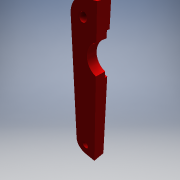
# Autodesk Inventor part: Carro XY_trava_A
Saved by Autodesk Inventor 2016 (Build 200138000, 138)
## iProperties
Created: 2016-08-11
Part Number: Carro XY_trava_A
Material: ABS Plastic
Document SubType Name: Modeling
Designer: Waldo
Density: 1.06 g/cm^3
Appearance: Smooth - White
Author: Waldo
Autodesk Inventor part; units mm, degrees
ref_plane "YZ Plane" through (0, 0, 0) normal (1, 0, 0) x (0, 1, 0)
ref_plane "XZ Plane" through (0, 0, 0) normal (0, 1, 0) x (-1, 0, 0)
ref_plane "XY Plane" through (0, 0, 0) normal (0, 0, 1) x (1, 0, 0)
sketch "Sketch1" plane through (0, 0, 0) normal (0, 1, 0) x (-1, 0, 0)
  line L0 (14.0376, 28.5915) -> (4.0376, 28.5915)
  line L1 (4.0376, 28.5915) -> (4.0376, -31.4085)
  line L2 (4.0376, -31.4085) -> (14.0376, -31.4085)
  line L3 (14.0376, -31.4085) -> (14.0376, 28.5915)
  point P0 (0, 0)
  dimension "d0" = 60
  dimension "d1" = 10
  constraints: 8 end point, 2 parallel, 1 horizontal, 1 perpendicular
  measures "d0" distance of L2.end L0.start
  measures "d1" distance of L0.start L0.end
extrude "Extrusion1" add sketch "Sketch1" along normal blind 5.2
sketch "Sketch2" plane through (0, 0, 0) normal (0, -1, 0) x (1, 0, 0)
  arc A0 (-14.0376, -26.4085) -> (-9.0376, -31.4085) centre (-9.0376, -26.4085) ccw projected
  arc A1 (-9.0376, 28.5915) -> (-14.0376, 23.5915) centre (-9.0376, 23.5915) ccw projected
  circle A2 centre (-9.0376, -26.4085) radius 1.5 projected
  circle A3 centre (-9.0376, 23.5915) radius 1.5 projected
  point P0 (0, 0)
fillet "Fillet1" radius 5 2 edges at (-14.0376, 2.6, -31.4085) (-14.0376, 2.6, 28.5915)
hole "Hole1" at (-9.0376, 0, -26.4085) at (-9.0376, 0, 23.5915) direction (0, 1, 0) diameter 3 end through all
sketch "Sketch3" plane through (0, 5.2, 0) normal (0, 1, 0) x (1, 0, 0)
  circle A0 centre (-2.0376, -12.5915) radius 7.9 projected
  point P0 (0, 0)
extrude "Extrusion2" cut sketch "Sketch3" against normal blind 1.1
sketch "Sketch4" plane through (0, 4.1, 0) normal (0, 1, 0) x (1, 0, 0)
  circle A0 centre (-2.0376, -12.5915) radius 4.5 projected
  circle A1 centre (24.4624, -12.0915) radius 6 projected
  circle A2 centre (24.4624, 14.9085) radius 6 projected
  circle A3 centre (-2.0376, 15.4085) radius 4.5 projected
  circle A4 centre (30.9624, -22.5915) radius 3 projected
  circle A5 centre (-9.0376, 26.4085) radius 3 projected
  circle A6 centre (30.9624, 25.4085) radius 3 projected
  circle A7 centre (-9.0376, -23.5915) radius 3 projected
  arc A8 (4.9041, -26.2279) -> (6.8708, -28.5915) centre (6.8708, -26.5915) ccw projected
  line L0 (6.8708, -28.5915) -> (30.9624, -28.5915) projected
  arc A9 (30.9624, -28.5915) -> (35.9624, -23.5915) centre (30.9624, -23.5915) ccw projected
  line L1 (35.9624, -23.5915) -> (35.9624, 1.4085) projected
  line L2 (35.9624, 1.4085) -> (35.9624, 26.4085) projected
  arc A10 (35.9624, 26.4085) -> (30.9624, 31.4085) centre (30.9624, 26.4085) ccw projected
  line L3 (30.9624, 31.4085) -> (6.8708, 31.4085) projected
  arc A11 (6.8708, 31.4085) -> (4.9041, 29.0448) centre (6.8708, 29.4085) ccw projected
  arc A12 (-1.9792, 29.0448) -> (4.9041, 29.0448) centre (1.4624, 28.4085) ccw projected
  arc A13 (-1.9792, 29.0448) -> (-3.9459, 31.4085) centre (-3.9459, 29.4085) ccw projected
  line L4 (-3.9459, 31.4085) -> (-9.0376, 31.4085) projected
  arc A14 (-9.0376, 31.4085) -> (-14.0376, 26.4085) centre (-9.0376, 26.4085) ccw projected
  line L5 (-14.0376, 26.4085) -> (-14.0376, 1.4085) projected
  line L6 (-14.0376, 1.4085) -> (-14.0376, -23.5915) projected
  arc A15 (-14.0376, -23.5915) -> (-9.0376, -28.5915) centre (-9.0376, -23.5915) ccw projected
  line L7 (-9.0376, -28.5915) -> (-3.9459, -28.5915) projected
  arc A16 (-3.9459, -28.5915) -> (-1.9792, -26.2279) centre (-3.9459, -26.5915) ccw projected
  arc A17 (4.9041, -26.2279) -> (-1.9792, -26.2279) centre (1.4624, -25.5915) ccw projected
  circle A18 centre (-2.0376, -12.5915) radius 5.5 projected
  circle A19 centre (-2.0376, -12.5915) radius 5.7
  point P0 (0, 0)
  dimension "d14" = 0.2
  constraints: 1 centre point
  measures "d14" radial gap between concentric circles of A18 A19
extrude "Extrusion3" cut sketch "Sketch4" against normal through all contours A0 | A18 | A19
body "Solid1"
